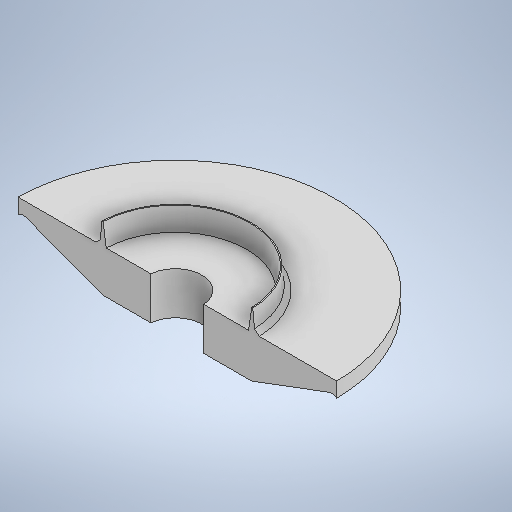
# Autodesk Inventor part: Wire Passthrough Resin Seal
Saved by Autodesk Inventor 2025 (Build 290162000, 162)
## iProperties
Created: 2025-10-24
Part Number: Wire Passthrough Resin Seal
Material: Generic
Document SubType Name: Modeling
Designer: mumin
Density: 1 g/cm^3
Appearance: Default
Author: mumin
Autodesk Inventor part; units mm, degrees
ref_plane "YZ Plane" through (0, 0, 0) normal (1, 0, 0) x (0, 1, 0)
ref_plane "XZ Plane" through (0, 0, 0) normal (0, 1, 0) x (-1, 0, 0)
ref_plane "XY Plane" through (0, 0, 0) normal (0, 0, 1) x (1, 0, 0)
sketch "Sketch1" plane through (0, 0, 0) normal (0, 1, 0) x (-1, 0, 0)
  circle A0 centre (0, 0) radius 1.25
  circle A1 centre (0, 0) radius 7.5
  dimension "d0" = 2.5
  dimension "d1" = 15
  constraints: 2 centre point, 2 coincident
  measures "d0" diameter of A0
  measures "d1" diameter of A1
extrude "Body" add sketch "Sketch1" along normal blind 2
chamfer "Bottom Chamfer" distance 1.5 distance2 4 1 edges at (7.5, 0, 0) measured on face at (-7.4757, 1.3333, -0.6035)
sketch "Sketch4" plane through (0, 0, 0) normal (1, 0, 0) x (0, 1, 0)
  line L0 (2, -7.5) -> (2, 7.5)
  line L1 (2, 3.35) -> (3, 3.35)
  line L2 (3, 3.35) -> (3, 3.65)
  line L3 (3, 3.65) -> (2, 3.65)
  line L4 (2, 3.65) -> (2, 3.35)
  line L5 (2, 3.65) -> (3, 3.55)
  line L6 (2, 3.65) -> (2.311367, 3.65) construction
  line L7 (3, 3.5) -> (2, 3.35)
  line L8 (-0.462273, 0) -> (2.77364, 0)
  point P0 (0, 0)
  point P1 (2, 0)
  point P2 (2, 3.65)
  dimension "d16" = 1
  dimension "d17" = 0.3
  dimension "d18" = 3.65
  dimension "d34" = 0.1
  constraints: 14 end point, 3 midpoint, 2 horizontal, 2 parallel, 2 point on line, 1 perpendicular
  measures "d16" distance of L3.end L2.end
  measures "d17" distance of L2.end L1.end
  measures "d18" distance from line of point (2, 0) L3
  measures "d34" distance of L2.end L5.end
revolve "Centering Lip" add sketch "Sketch4" angle 360 about axis through (0, -10, 0) along (0, 1, 0) contours L0 L5 L2 L7
sketch "Sketch6" plane through (0, 0, 0) normal (0, 0, 1) x (1, 0, 0)
  line L0 (7.5, 2) -> (-7.5, 2) projected
  line L1 (7.5, 2) -> (7.2, 2)
  line L2 (7.2, 2) -> (7.2, 1.3)
  line L3 (7.2, 1.3) -> (7.5, 1.3)
  line L4 (7.5, 1.3) -> (7.5, 2)
  line L5 (-7.5, 1.5) -> (7.5, 1.5) projected
  line L6 (7.5, 1.3) -> (7.2, 1.5)
  line L7 (0, -0.4) -> (0, 2.4) projected
  point P0 (0, 0)
  dimension "d27" = 0.3
  dimension "d28" = 0.7
  constraints: 10 end point, 2 parallel, 2 point on line, 1 horizontal, 1 perpendicular
  measures "d27" distance between parallel lines of L4 L2
  measures "d28" distance of L0.start L3.end
revolve "Revolution2" add sketch "Sketch6" angle 360 about axis through (0, -10, 0) along (0, 1, 0) contours L4 L6 L5
fillet "Fillet1" radius 0.3 2 edges at (0, 1.428, 7.308) (0, 1.428, -7.308)
sketch "Sketch7" plane through (0, 0, 0) normal (0, -1, 0) x (1, 0, 0)
  line L0 (-7.5, -0.1) -> (7.5, -0.1)
  line L1 (7.5, -0.1) -> (7.5, 7.5)
  line L2 (7.5, 7.5) -> (-7.5, 7.5)
  line L3 (-7.5, 7.5) -> (-7.5, -0.1)
  circle A0 centre (0, 0) radius 7.5 projected
  point P0 (-7.499333, -0.1)
  point P1 (7.499333, -0.1)
  dimension "d31" = 0.1
  constraints: 8 end point, 3 tangent, 2 parallel, 1 horizontal, 1 perpendicular
  measures "d31" distance from line of L0 point (0, 0)
sketch "Sketch7 outline for Extrusion5" plane through (0, 0, 0) normal (0, -1, 0) x (1, 0, 0)
  arc A0 (7.499333, -0.1) -> (-7.499333, -0.1) centre (0, 0) ccw
  line L0 (-7.499333, -0.1) -> (7.499333, -0.1)
extrude "Extrusion5" cut sketch "Sketch7 outline for Extrusion5" against normal through all
chamfer "Chamfer3" distance 0.2 angle 45 1 edges at (0, 2, -3.65)
body "Solid1"
